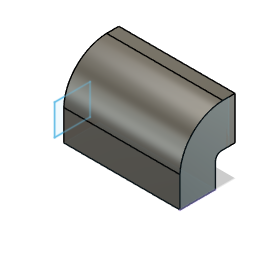
Inverter_fan_cabinet_curved (Autodesk Fusion 360 design; units mm, degrees)
Autodesk Fusion 360 part; units mm, degrees
sketch "Sketch1" plane through (0, 0, 0) normal (0, 1, 0) x (1, 0, 0)
  line L0 (15, -10) -> (205, -10)
  line L1 (205, -10) -> (205, -80)
  line L2 (205, -80) -> (15, -80)
  line L3 (15, -80) -> (15, -10)
  dimension "d1" = 190
  dimension "d2" = 70
  constraint horizontal L0
  constraint vertical L1
  constraint horizontal L2
  constraint vertical L3
  measures "d1" distance of L0.start L0.end
  measures "d2" distance of L0.start L2.end
extrude "Extrude1" add sketch "Sketch1" along normal blind 70
ref_plane "WorkPlane1" through (110, 35, 150) normal (0, 0, 1) x (1, 0, 0)
sketch "Sketch2" plane through (15, 0, 0) normal (-1, 0, 0) x (0, 0, 1)
  line L0 (10, 0) -> (80, 0)
  line L1 (80, 0) -> (80, 70)
  line L2 (80, 70) -> (10, 70)
  line L3 (10, 70) -> (10, 0)
  arc A0 (80, 0) -> (10, 70) centre (7.6705, -2.3295) ccw
  constraint coincident L0.end L1.start
  constraint coincident L2.end L3.start
extrude "Extrude2" cut sketch "Sketch2" against normal blind 220 contours L1 L2 A0
sketch "Sketch3" plane through (0, 0, 0) normal (1, 0, 0) x (0, 0, -1)
  line L0 (-80, 0) -> (-22, 0)
  line L1 (-22, 0) -> (-22, -50)
  line L2 (-22, -50) -> (-80, -50)
  line L3 (-80, -50) -> (-80, 0)
  dimension "d8" = 58
  dimension "d9" = 50
  constraint horizontal L0
  constraint vertical L1
  constraint horizontal L2
  constraint vertical L3
  measures "d8" distance of L0.start L0.end
  measures "d9" distance of L0.start L2.end
sketch "Sketch4" plane through (0, 0, 0) normal (0, -1, 0) x (1, 0, 0)
  line L0 (205, 80) -> (15, 80)
  line L1 (15, 80) -> (15, 10)
  line L2 (15, 10) -> (205, 10)
  line L3 (205, 10) -> (205, 80)
  line L4 (15, 80) -> (205, 80)
  line L5 (205, 80) -> (205, 22)
  line L6 (205, 22) -> (15, 22)
  line L7 (15, 22) -> (15, 80)
  dimension "d10" = 190
  dimension "d11" = 58
  constraint horizontal L4
  constraint vertical L5
  constraint horizontal L6
  constraint vertical L7
  constraint coincident L0.end L1.start
  measures "d10" distance of L0.end L0.start
  measures "d11" distance of L0.end L6.end
extrude "Extrude3" add sketch "Sketch4" along normal blind 50 contours L0 L1 L3 L4 L5 L6 L7
sketch "Sketch5" plane through (0, 0, 10) normal (0, 0, -1) x (-1, 0, 0)
  line L0 (-205, 0) -> (-15, 0)
  line L1 (-15, 0) -> (-15, 70)
  line L2 (-15, 70) -> (-205, 70)
  line L3 (-205, 70) -> (-205, 0)
sketch "Sketch6" plane through (0, -50, 0) normal (0, -1, 0) x (1, 0, 0)
  line L0 (15, 22) -> (205, 22)
  line L1 (205, 22) -> (205, 80)
  line L2 (205, 80) -> (15, 80)
  line L3 (15, 80) -> (15, 22)
sketch "Sketch7" plane through (0, 0, 10) normal (0, 0, -1) x (-1, 0, 0)
extrude "Extrude4" add sketch "Sketch5" along normal blind 10
fillet "Fillet2" radius 10 1 edges at (110, 0, 22)
sketch "Sketch9" plane through (205, 0, 0) normal (1, 0, 0) x (0, 0, -1)
  arc A0 (-10, 70) -> (-80, 0) centre (-7.6705, -2.3295) ccw
  line L0 (-80, 0) -> (-80, -50)
  line L1 (-22, -50) -> (-22, -10)
  arc A1 (-12, 0) -> (-22, -10) centre (-12, -10) ccw
  line L2 (-12, 0) -> (0, 0)
  line L3 (0, 0) -> (0, 70)
  line L4 (0, 70) -> (-10, 70)
  line L5 (-80, -50) -> (-22, -50)
sketch "Sketch10" plane through (205, 0, 0) normal (1, 0, 0) x (0, 0, -1)
extrude "Extrude6" add 1 faces at (141.6667, 46.6667, 0) along direction (0, 0, -1) blind 10
shell "Shell3" thickness 5 removed faces 1 at (78.3333, -50, 60.6667)
sketch "Sketch11" plane through (0, 0, -10) normal (0, 0, -1) x (-1, 0, 0)
  line L0 (-205, 70) -> (-205, 0)
  line L1 (-205, 0) -> (-15, 0)
  line L2 (-15, 0) -> (-15, 70)
  line L3 (-15, 70) -> (-205, 70)
  circle A0 centre (-169.8496, 35) radius 25
  circle A1 centre (-109.8496, 35) radius 25
  circle A2 centre (-49.8496, 35) radius 25
  dimension "d37" = 50
  dimension "d38" = 50
  dimension "d39" = 50
  dimension "d40" = 35.1504
  dimension "d41" = 60
  dimension "d42" = 60
  dimension "d43" = 35
  dimension "d44" = 35
  dimension "d45" = 35
  measures "d37" diameter of A0
  measures "d38" diameter of A1
  measures "d39" diameter of A2
  measures "d40" distance of L0 A0.centre
  measures "d41" horizontal distance of A0.centre A1.centre
  measures "d42" horizontal distance of A1.centre A2.centre
  measures "d43" distance of L3 A1.centre
  measures "d44" distance of L3 A2.centre
  measures "d45" distance of L3 A0.centre
extrude "Extrude7" cut sketch "Sketch11" against normal blind 10 contours A0 | A1 | A2
